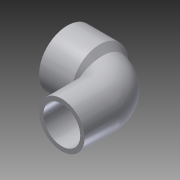
# Autodesk Inventor part: 2 Way .75 to 1 thread
Saved by Autodesk Inventor 2013 (Build 170138000, 138)
## iProperties
Created: 2013-06-27
Part Number: 2 Way .75 to 1 thread
Material: PVC-Piping
Document SubType Name: Modeling
Designer: Kyle
Density: 1 g/cm^3
Author: Kyle
Autodesk Inventor part; units mm, degrees
sketch "Sketch1" plane through (0, 0, 0) normal (0, 0, 1) x (1, 0, 0)
  circle A0 centre (0, 0) radius 10.795
  circle A1 centre (0, 0) radius 13.335
  line L0 (-13.335, 13.335) -> (-13.335, -13.335)
  line L1 (-13.335, 13.335) -> (13.335, 13.335)
  dimension "d0" = 21.59
  dimension "d2" = 26.67
  constraints: 4 end point, 2 centre point, 2 tangent, 1 coincident, 1 perpendicular, 1 vertical
  measures "d0" diameter of A0
  measures "d2" diameter of A1
ref_plane "Work Plane1" through (-13.335, 13.335, 0) normal (1, 0, 0) x (0, 1, 0)
sketch "Sketch2" plane through (-13.335, 13.335, 0) normal (1, 0, 0) x (0, 1, 0)
  circle A0 centre (-13.335, -16.51) radius 16.51
  circle A1 centre (-13.335, -16.51) radius 13.335
  line L0 (-26.67, -33.02) -> (3.175, -33.02)
  line L1 (3.175, -33.02) -> (3.175, -3.175)
  point P0 (-13.335, 0)
  dimension "d3" = 33.02
  dimension "d5" = 16.51
  dimension "d6" = 26.67
  constraints: 4 end point, 2 centre point, 2 tangent, 1 horizontal, 1 perpendicular
  measures "d3" diameter of A0
  measures "d5" distance of point (-13.335, 0) A0.centre
  measures "d6" diameter of A1
extrude "Extrusion1" add sketch "Sketch2" against normal blind 19.05 contours A0
extrude "Extrusion2" add sketch "Sketch1" along normal blind 19.05 contours A1
sketch "Sketch3" plane through (-13.335, 13.335, 0) normal (1, 0, 0) x (0, 0, -1)
  circle A0 centre (16.51, -13.335) radius 13.335 projected
  arc A1 (0, -13.335) -> (16.51, 3.175) centre (16.51, -13.335) ccw projected
  arc A2 (16.51, 3.175) -> (0, -13.335) centre (16.51, -13.335) ccw projected
sketch "Sketch4" plane through (0, 0, 0) normal (0, 0, -1) x (-1, 0, 0)
  circle A0 centre (0, 0) radius 10.795 projected
  arc A1 (-13.335, 0) -> (13.335, 0) centre (0, 0) ccw projected
  arc A2 (13.335, 0) -> (-13.335, 0) centre (0, 0) ccw projected
ref_plane "Work Plane2" through (0, 0, 0) normal (0, 1, 0) x (0, 0, 1)
sketch "Sketch5" plane through (0, 0, 0) normal (0, 1, 0) x (0, 0, 1)
  arc A0 (0, 0) -> (-16.7206, -13.0978) centre (-0.7794, -16.2266) ccw
  constraints: 2 point on circle, 1 centre point
sweep "Sweep1" add profiles "Sketch4" path "Sketch5"
ref_plane "Work Plane3" through (-6.985, 0, -16.51) normal (1, 0, 0) x (0, 0, -1)
sketch "Sketch6" plane through (-6.985, 0, -16.51) normal (1, 0, 0) x (0, 0, -1)
  circle A0 centre (0, 0) radius 10.795
  circle A1 centre (0, 0) radius 8.255
  point P0 (-16.51, 0)
  dimension "d14" = 21.59
  dimension "d16" = 16.51
  constraints: 2 centre point
  measures "d14" diameter of A0
  measures "d16" diameter of A1
loft "Loft1" add profiles "Sketch6" section 1 edges at (-13.335, 11.6743, -4.8357) (-13.335, -11.6743, -28.1843) contours A0 | A1
thread "Thread1" size "1 1/16-8 UNC" class "2B" standard "ANSI Unified Screw Threads" full length
body "Solid1"
